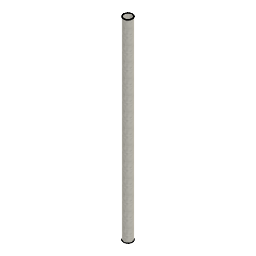
Antenna Assembly (Autodesk Fusion 360 archive; units mm, degrees)
design "GFK Rod"
part number: 2026-07-02-19-40-21-318
Autodesk Fusion 360 part; units mm, degrees
(part 1 of 2)
sketch "Skizze1" plane through (0, 0, 0) normal (0, 0, 1) x (1, 0, 0)
  circle A0 centre (0, 0) radius 14
  circle A1 centre (0, 0) radius 15.5
  dimension "d1" = 28
  dimension "d2" = 31
  constraint coincident A0.centre A1.centre
  measures "d1" diameter of A0
  measures "d2" diameter of A1
extrude "Extrusion1" add sketch "Skizze1" along normal blind 521.6482 and the other way blind 150
equation "d3 = 40 mm + ( 13.25 * 36.2376 ) * 1 mm + 4.5 mm - 3 mm"
named bodies: "GFK Rod"

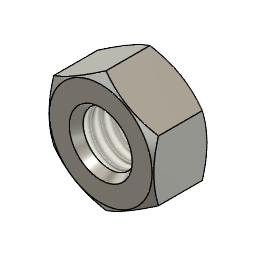
design "Sechskantmutter, normale Form ISO 4032 - M6 Stahl 6 Einfach"
description: Sechskantmutter, normale Form ISO 4032 - M6
part number: ISO 4032 - M6 Stahl 6 Einfach
Autodesk Fusion 360 part; units mm, degrees
sketch "Sketch1" plane through (0, 0, 0) normal (0, 1, 0) x (1, 0, 0)
  line L0 (0, 0) -> (0, -5.2)
  line L1 (-3, 0) -> (-4.9, 0)
  line L2 (-4.9, 0) -> (-5.775, -0.5052)
  line L3 (-5.775, -0.5052) -> (-5.775, -4.6948)
  line L4 (-5.775, -4.6948) -> (-4.9, -5.2)
  line L5 (-4.9, -5.2) -> (-3, -5.2)
  line L6 (-3, -5.2) -> (-3, 0)
  dimension "d121" = 6
  dimension "d122" = 30
  dimension "d123" = 30
  dimension "d128" = 11.55
  dimension "d172" = 9.8
  dimension "d179" = 5.2
  constraint vertical L0
  constraint coincident L0 L0.end
  constraint coincident origin L0
  constraint horizontal L1
  constraint coincident L0.start L1
  constraint coincident L0.start origin
  constraint coincident L0.end L5
  constraint vertical L1.end L4.end
  measures "d122" angle of L1 L2
  measures "d123" angle of L4 L5
  measures "d179" distance of L1 L5
revolve "Revolve1" add sketch "Sketch1" angle 360 about axis through (0, 0, 0) along (0, 0, 1)
sketch "Sketch8" plane through (0, 0, 5.2) normal (0, 0, 1) x (1, 0, 0)
  line L0 (-5, -2.8897) -> (-5, 2.8897)
  circle A0 centre (0, 0) radius 3
  circle A1 centre (0, 0) radius 5.775
  dimension "d114" = 5
  constraint coincident L0.end A1
  constraint coincident L0.start A1
  constraint vertical L0
  measures "d114" distance of A0.centre L0
extrude "Extrude5" cut sketch "Sketch8" against normal blind 5.2 contours L0 A1 picked at (-5.125, -0.7039)
pattern_circular "C-Pattern2" count 6 over 360 about axis through (0, 0, 1.75) along (0, 0, 1) of "Extrude5"
thread "Thread3" "ISO Metric profile 6.0 M6x1 M6x1 6H" major diameter 6.147 minor diameter 5.035 pitch 1 angle 60 resizes the face on face at (-2.9963, 0.1495, 3.4667)
sketch "Sketch12" plane through (0, 0, 0) normal (0, 1, 0) x (1, 0, 0)
  line L0 (-3, 0) -> (0, 0)
  line L1 (-1.4989, -2.6) -> (-3, 0)
  line L2 (-3, -5.2) -> (0, -5.2)
  line L3 (-1.4989, -2.6) -> (-3, -5.2)
  line L4 (0, 0) -> (0, -5.2)
  dimension "d169" = 60
  dimension "d177" = 3
  dimension "d178" = 60
  constraint horizontal L0
  constraint coincident L1.start L3.start
  constraint vertical L0.start L2.start
  constraint coincident L2.end L4.end
  constraint coincident L0.end L4.start
  constraint perpendicular L2 L4
  measures "d169" angle of L2 L3
  measures "d177" distance of L0.start L4
  measures "d178" angle of L0 L1
revolve "Revolve3" cut sketch "Sketch12" angle 360 about axis through (0, 0, 1.75) along (0, 0, 1)
equation "adsk_nheig = 5.20 mm"
equation "adsk_maxdia = 11.55 mm"
equation "adsk_nomdia = 6.00 mm"
equation "d89 = -adsk_nheig"
equation "adsk_waflat = 10.00 mm"
equation "d114 = adsk_waflat / 2"
equation "adsk_chamang1 = 30.00 deg"
equation "adsk_chamang2 = 30.00 deg"
equation "d121 = adsk_nomdia"
equation "d122 = adsk_chamang1"
equation "d123 = adsk_chamang2"
equation "d128 = adsk_maxdia"
equation "d163 = adsk_nheig"
equation "adsk_beardia = 9.80 mm"
equation "d172 = adsk_beardia"
equation "d177 = adsk_nomdia * 0.5"
equation "d179 = adsk_nheig"

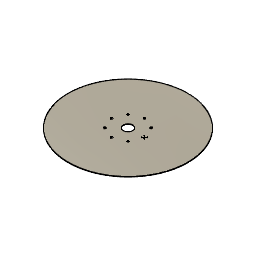
design "Aluminum Reflector"
part number: 2026-07-02-19-35-45-000
Autodesk Fusion 360 part; units mm, degrees
sketch "Skizze1" plane through (0, 0, 0) normal (0, 0, 1) x (1, 0, 0)
  circle A0 centre (0, 0) radius 200
  circle A1 centre (0, 0) radius 15.7
  circle A2 centre (0, 0) radius 54.873
  line L0 (50.553, -4.32) -> (50.553, 4.32)
  circle A3 centre (50.553, -4.32) radius 1.3
  circle A4 centre (59.193, -4.32) radius 1.3
  line L1 (50.553, -4.32) -> (59.193, 4.32) construction
  line L2 (50.553, 4.32) -> (59.193, 4.32)
  line L3 (59.193, -4.32) -> (50.553, 4.32) construction
  line L4 (59.193, 4.32) -> (59.193, -4.32)
  circle A5 centre (50.553, 4.32) radius 1.3
  circle A6 centre (54.873, 0) radius 2.25
  line L5 (59.193, -4.32) -> (50.553, -4.32)
  circle A7 centre (59.193, 4.32) radius 1.3
  circle A8 centre (-54.873, 0) radius 3.1
  circle A9 centre (38.8011, 38.8011) radius 3.1
  circle A10 centre (0, 54.873) radius 3.1
  circle A11 centre (-38.8011, 38.8011) radius 3.1
  circle A12 centre (-38.8011, -38.8011) radius 3.1
  circle A13 centre (0, -54.873) radius 3.1
  circle A14 centre (38.8011, -38.8011) radius 3.1
  point P0 (54.873, 0)
  point P1 (54.873, 0)
  dimension "d1" = 400
  dimension "d2" = 31.4
  dimension "d3" = 109.746
  dimension "d6" = 4.5
  dimension "d7" = 8.64
  dimension "d8" = 8.64
  dimension "d9" = 2.6
  dimension "d10" = 2.6
  dimension "d11" = 2.6
  dimension "d12" = 2.6
  dimension "d13" = 6.2
  dimension "d15" = 270
  constraint coincident A0.centre A1.centre
  constraint concentric A0 A1
  constraint coincident P1 P0
  constraint horizontal L5
  constraint perpendicular L0 L5
  constraint parallel L2 L5
  constraint parallel L0 L4
  constraint coincident P1 L3
  constraint coincident P1 L1
  constraint coincident L1.end L2.end
  constraint coincident A4.centre L3.start
  constraint coincident L0.end L2.start
  constraint coincident L0.start A3.centre
  constraint coincident A2 P1
  constraint horizontal A0.centre P1
  constraint coincident A2 A8.centre
  measures "d1" diameter of A0
  measures "d2" diameter of A1
  measures "d3" diameter of A2
  measures "d6" diameter of A6
  measures "d7" distance of L0.end L1.end
  measures "d8" distance of L0.end L0.start
  measures "d9" diameter of A7
  measures "d10" diameter of A4
  measures "d11" diameter of A5
  measures "d12" diameter of A3
  measures "d13" diameter of A8
extrude "Extrusion1" add sketch "Skizze1" along normal blind 1.5 contours A0 | A2 L0 A3 L2 A5 A6 L5 | A2 A4 L2 L4 A6 L5 A7 | A2 L0 A3 L2 A5 L5 A8 A9 A10 A11 A12 A13 A14
named bodies: "Aluminum Reflector"

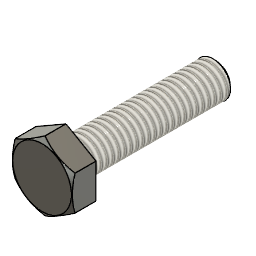
design "Sechskantschraube mit Ganzgewinde DIN EN 24018 - M6 x 25 Stahl 4.6 Einfach"
description: Sechskantschraube mit Ganzgewinde DIN EN 24018 - M6 x 25
part number: DIN EN 24018 - M6 x 25 Stahl 4.6 Einfach
Autodesk Fusion 360 part; units mm, degrees
sketch "Sketch1" plane through (0, 0, 0) normal (0, 1, 0) x (1, 0, 0)
  line L0 (-3, 0) -> (-3, 25)
  line L1 (-3, 25) -> (0, 25)
  line L2 (0, 25) -> (0, -4)
  line L3 (-3, 0) -> (-5.775, 0)
  line L4 (-5.775, 0) -> (-5.775, -3.4948)
  line L5 (-4.9, -4) -> (0, -4)
  line L6 (-5.775, -3.4948) -> (-4.9, -4)
  dimension "d81" = 11.55
  dimension "d135" = 6
  dimension "d137" = 4
  dimension "d138" = 25
  dimension "d153" = 30
  dimension "d154" = 9.8
  constraint perpendicular L0 L1
  constraint perpendicular L0 L3
  constraint coincident origin L3
  constraint vertical L2
  constraint coincident L2 L5.end
  constraint perpendicular L2 L5
  constraint coincident L0.start L3.start
  constraint coincident L0.end L1.start
  constraint coincident origin L2
  constraint vertical L4
  measures "d137" distance of L3 L5
  measures "d138" distance of L1 L3
  measures "d153" angle of L5 L6
revolve "Revolve1" add sketch "Sketch1" angle 360 about axis through (0, 0, -25) along (0, 0, 1)
sketch "Sketch8" plane through (0, 0, 0) normal (0, 0, 1) x (1, 0, 0)
  line L0 (-5, -2.8868) -> (0, -5.7735)
  line L1 (0, -5.7735) -> (5, -2.8868)
  line L2 (5, -2.8868) -> (5, 2.8868)
  line L3 (5, 2.8868) -> (0, 5.7735)
  line L4 (0, 5.7735) -> (-5, 2.8868)
  line L5 (-5, 2.8868) -> (-5, -2.8868)
  circle A0 centre (0, 0) radius 5.8
  dimension "d160" = 10
  dimension "d161" = 11.6
  constraint vertical L5
  constraint coincident A0.centre origin
  measures "d160" distance of L2 L5
  measures "d161" diameter of A0
extrude "Extrude5" cut sketch "Sketch8" along normal through all
thread "Thread3" "ISO Metric profile 6.0 M6x1 M6x1 6g" major diameter 5.884 minor diameter 4.7435 pitch 1 angle 60 resizes the face on face at (-2.9851, 0.2987, -8.3333) from (0, 0, -1) to (0, 0, -25)
sketch "Sketch13" plane through (0, 0, 0) normal (0, 1, 0) x (1, 0, 0)
  line L0 (0, 25) -> (0, -4)
  line L1 (0, 25) -> (-3.06, 25)
  line L2 (-3.06, 25) -> (-3.06, 24.3865)
  line L3 (-3.06, 24.3865) -> (-2.3866, 25)
  dimension "d155" = 0.6135
  dimension "d156" = 2.3866
  dimension "d157" = 3.06
  constraint coincident L0.start L1.start
  constraint perpendicular L0 L1
  constraint perpendicular L1 L2
  constraint coincident L1 L3.end
  measures "d155" distance of L1 L2.end
  measures "d156" distance of L0 L3.end
  measures "d157" distance of L0.start L2
revolve "Revolve4" cut sketch "Sketch13" angle 360 about axis through (0, 0, 1.75) along (0, 0, 1)
equation "adsk_nomlen = 25.00 mm"
equation "adsk_headh = 4.00 mm"
equation "adsk_headdia = 11.55 mm"
equation "adsk_nomdia = 6.00 mm"
equation "d81 = adsk_headdia"
equation "adsk_waflat = 10.00 mm"
equation "adsk_thrlen = 24.00 mm"
equation "adsk_chamang2 = 30.00 deg"
equation "d135 = adsk_nomdia"
equation "d137 = adsk_headh"
equation "d138 = adsk_nomlen"
equation "adsk_endpointdia = 4.7731 mm"
equation "adsk_startlen = 0.61345 mm"
equation "d153 = adsk_chamang2"
equation "d154 = adsk_waflat * 0.98"
equation "d155 = adsk_startlen"
equation "d156 = adsk_endpointdia / 2"
equation "d157 = adsk_nomdia * 0.51"
equation "d159 = min(adsk_thrlen; adsk_nomlen - 0.001 mm)"
equation "d160 = adsk_waflat"
equation "d161 = max(adsk_waflat * 1.16; adsk_headdia)"

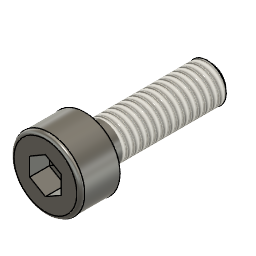
design "Zylinderschraube mit gestanztem Innensechskant ANSI B18.3.1M - M2.5x0.45 x 8 Stahlklasse 2 Einfach"
description: Zylinderschraube mit gestanztem Innensechskant ANSI B18.3.1M - M2.5x0.45 x 8
part number: BSHCS ANSI B18.3.1M - M2.5x0.45 x 8 Stahlklasse 2 Einfach
Autodesk Fusion 360 part; units mm, degrees
sketch "Sketch1" plane through (0, 0, 0) normal (0, 1, 0) x (1, 0, 0)
  line L0 (-1.25, 0) -> (-1.25, 8)
  line L1 (-1.25, 8) -> (0, 8)
  line L2 (0, 8) -> (0, -2.5)
  line L3 (-1.25, 0) -> (-2.25, 0)
  line L4 (-2.25, 0) -> (-2.25, -2.5)
  line L5 (-2.25, -2.5) -> (0, -2.5)
  dimension "d101" = 8
  dimension "d102" = 2.5
  dimension "d109" = 4.5
  dimension "d110" = 2.5
  constraint perpendicular L0 L1
  constraint collinear origin L1.end L2.end
  constraint perpendicular L0 L3
  constraint coincident origin L3
  constraint vertical L2
  constraint coincident L2 L5.end
  constraint perpendicular L2 L5
  measures "d101" distance of origin L1
  measures "d102" distance of L3.end L5
revolve "Revolve1" add sketch "Sketch1" angle 360 about axis through (0, 0, -8) along (0, 0, 1)
ref_plane "WorkPlane1" through (0, 0, 2.5) normal (0, 0, 1) x (1, 0, 0)
sketch "Sketch6" plane through (0, 0, 2.5) normal (0, 0, 1) x (1, 0, 0)
  line L0 (0, -1.1547) -> (1, -0.5774)
  line L1 (1, -0.5774) -> (1, 0.5774)
  line L2 (1, 0.5774) -> (0, 1.1547)
  line L3 (0, 1.1547) -> (-1, 0.5774)
  line L4 (-1, 0.5774) -> (-1, -0.5774)
  line L5 (-1, -0.5774) -> (0, -1.1547)
  dimension "d111" = 2
  constraint vertical L1
  measures "d111" distance of L1 L4
extrude "Extrude1" cut sketch "Sketch6" against normal blind 1.25
extrude "Extrude2" cut 1 faces at (-0.3333, -0.1925, 1.25) along direction (0, 0, -1) blind 1.25 draft -85
thread "Thread3" "ANSI Metric M Profile 2.5 M2.5x0.45 M2.5x0.45 4g6g" major diameter 2.43 minor diameter 1.9295 pitch 0.45 angle 60 resizes the face on face at (-1.2438, 0.1245, -5.3333) from (0, 0, -1.1761) to (0, 0, -8)
fillet "Fillet4" radius 0.25 1 edges at (-2.0977, 0.8136, 2.5)
sketch "Sketch7" plane through (0, 0, 0) normal (0, 1, 0) x (1, 0, 0)
  line L0 (-1.275, 8) -> (-1.275, 7.7239)
  line L1 (-1.275, 7.7239) -> (-0.9739, 8)
  line L2 (0, 8) -> (0, -2.5)
  line L3 (-1.275, 8) -> (0, 8)
  dimension "d104" = 0.9739
  dimension "d105" = 1.275
  dimension "d106" = 0.2761
  constraint coincident L2.start L3.end
  constraint perpendicular L2 L3
  constraint coincident L1.end L3
  constraint perpendicular L0 L3
  measures "d104" distance of L1.end L2
  measures "d105" distance of L0 L2.start
  measures "d106" distance of L0.end L3
revolve "Revolve3" cut sketch "Sketch7" angle 360 about axis through (0, 0, 1.75) along (0, 0, 1)
equation "adsk_nomlen = 8.00 mm"
equation "adsk_headh = 2.50 mm"
equation "adsk_headdia = 4.50 mm"
equation "adsk_nomdia = 2.50 mm"
equation "adsk_philwidth = 2.00 mm"
equation "d31 = -adsk_phildepth"
equation "adsk_phildepth = 1.25 mm"
equation "d71 = adsk_headh"
equation "d76 = -adsk_phildepth"
equation "adsk_thrlen = 6.8239475 mm"
equation "d86 = adsk_nomdia * 0.1"
equation "adsk_startlen = 0.276053 mm"
equation "adsk_endpointdia = 1.947895 mm"
equation "d101 = adsk_nomlen"
equation "d102 = adsk_headh"
equation "d104 = adsk_endpointdia / 2"
equation "d105 = adsk_nomdia * 0.51"
equation "d106 = adsk_startlen"
equation "d108 = min(adsk_thrlen; adsk_nomlen - 0.001 mm)"
equation "d109 = adsk_headdia"
equation "d110 = adsk_nomdia"
equation "d111 = adsk_philwidth"

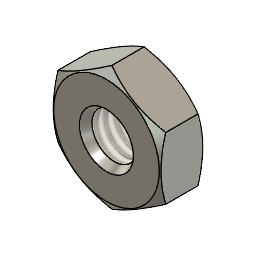
design "Sechskantmutter, normale Form DIN 970 - M2.5 Stahl 6 Einfach"
description: Sechskantmutter, normale Form DIN 970 - M2.5
part number: DIN 970 - M2.5 Stahl 6 Einfach
Autodesk Fusion 360 part; units mm, degrees
sketch "Sketch1" plane through (0, 0, 0) normal (0, 1, 0) x (1, 0, 0)
  line L0 (0, 0) -> (0, -2)
  line L1 (-1.25, 0) -> (-2.45, 0)
  line L2 (-2.45, 0) -> (-2.8875, -0.2526)
  line L3 (-2.8875, -0.2526) -> (-2.8875, -1.7474)
  line L4 (-2.8875, -1.7474) -> (-2.45, -2)
  line L5 (-2.45, -2) -> (-1.25, -2)
  line L6 (-1.25, -2) -> (-1.25, 0)
  dimension "d121" = 2.5
  dimension "d122" = 30
  dimension "d123" = 30
  dimension "d128" = 5.775
  dimension "d172" = 4.9
  dimension "d179" = 2
  constraint vertical L0
  constraint coincident L0 L0.end
  constraint coincident origin L0
  constraint horizontal L1
  constraint coincident L0.start L1
  constraint coincident L0.start origin
  constraint coincident L0.end L5
  constraint vertical L1.end L4.end
  measures "d122" angle of L1 L2
  measures "d123" angle of L4 L5
  measures "d179" distance of L1 L5
revolve "Revolve1" add sketch "Sketch1" angle 360 about axis through (0, 0, 0) along (0, 0, 1)
sketch "Sketch8" plane through (0, 0, 2) normal (0, 0, 1) x (1, 0, 0)
  line L0 (-2.5, -1.4449) -> (-2.5, 1.4449)
  circle A0 centre (0, 0) radius 1.25
  circle A1 centre (0, 0) radius 2.8875
  dimension "d114" = 2.5
  constraint coincident L0.end A1
  constraint coincident L0.start A1
  constraint vertical L0
  measures "d114" distance of A0.centre L0
extrude "Extrude5" cut sketch "Sketch8" against normal blind 2 contours L0 A1 picked at (-2.5625, 0.3519)
pattern_circular "C-Pattern2" count 6 over 360 about axis through (0, 0, 1.75) along (0, 0, 1) of "Extrude5"
thread "Thread3" "ISO Metric profile 2.5 M2.5x0.45 M2.5x0.45 6H" major diameter 2.58 minor diameter 2.0755 pitch 0.45 angle 60 resizes the face on face at (-1.2438, 0.1245, 1.3333)
sketch "Sketch12" plane through (0, 0, 0) normal (0, 1, 0) x (1, 0, 0)
  line L0 (-1.25, 0) -> (0, 0)
  line L1 (-0.6726, -1) -> (-1.25, 0)
  line L2 (-1.25, -2) -> (0, -2)
  line L3 (-0.6726, -1) -> (-1.25, -2)
  line L4 (0, 0) -> (0, -2)
  dimension "d169" = 60
  dimension "d177" = 1.25
  dimension "d178" = 60
  constraint horizontal L0
  constraint coincident L1.start L3.start
  constraint vertical L0.start L2.start
  constraint coincident L2.end L4.end
  constraint coincident L0.end L4.start
  constraint perpendicular L2 L4
  measures "d169" angle of L2 L3
  measures "d177" distance of L0.start L4
  measures "d178" angle of L0 L1
revolve "Revolve3" cut sketch "Sketch12" angle 360 about axis through (0, 0, 1.75) along (0, 0, 1)
equation "adsk_nheig = 2.00 mm"
equation "adsk_maxdia = 5.775 mm"
equation "adsk_nomdia = 2.50 mm"
equation "d89 = -adsk_nheig"
equation "adsk_waflat = 5.00 mm"
equation "d114 = adsk_waflat / 2"
equation "adsk_chamang1 = 30.00 deg"
equation "adsk_chamang2 = 30.00 deg"
equation "d121 = adsk_nomdia"
equation "d122 = adsk_chamang1"
equation "d123 = adsk_chamang2"
equation "d128 = adsk_maxdia"
equation "d163 = adsk_nheig"
equation "adsk_beardia = 4.90 mm"
equation "d172 = adsk_beardia"
equation "d177 = adsk_nomdia * 0.5"
equation "d179 = adsk_nheig"

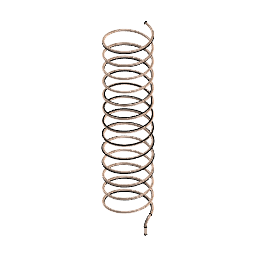
design "Copper Wire"
part number: 2026-07-02-19-25-43-179
Autodesk Fusion 360 part; units mm, degrees
coil "Grundkörper Spirale1" add diameter 109.746 section triangle out size 6 inside turns 13.25 pitch 36.2376 right hand placed x (1, 0, 0) y (0, 1, 0) z (0, 0, 1) at (0, 0, 0) makes body 1
sketch "Skizze2" plane through (0, 0, 0) normal (0, 0, 1) x (1, 0, 0)
  line L0 (54.873, 0, 0) -> (54.873, 0, -20)
  line L1 (54.873, 0, -20) -> (54.873, 0, -40)
  line L2 (54.873, 0, 0) -> (51.2639, 19.5586, 2.1021)
  spline S0 degree 3 poles (51.2639, 19.5586, 2.1021) (50.4481, 21.7028, 2.3432) (49.4982, 23.7958, 2.5844) (48.4186, 25.8203, 2.8255) (44.2021, 33.727, 3.7673) (38.0152, 40.5732, 4.7091) (30.5744, 45.5659, 5.6509) (23.1337, 50.5585, 6.5927) (14.4534, 53.6883, 7.5345) (5.5388, 54.5927, 8.4763) (-3.3756, 55.4972, 9.418) (-12.5073, 54.1747, 10.3598) (-20.7988, 50.7785, 11.3015) (-29.0901, 47.3824, 12.2432) (-36.5255, 41.9191, 13.1849) (-42.2439, 35.0214, 14.1267) (-47.9622, 28.1239, 15.0683) (-51.9527, 19.8051, 16.01) (-53.7534, 11.0283, 16.9517) (-55.554, 2.2518, 17.8934) (-55.1615, -6.966, 18.8351) (-52.6213, -15.5576, 19.7767) (-50.0813, -24.1491, 20.7184) (-45.3985, -32.0981, 21.66) (-39.1152, -38.4844, 22.6016) (-32.8321, -44.8705, 23.5432) (-24.9605, -49.6818, 24.4848) (-16.4118, -52.3612, 25.4264) (-7.8634, -55.0406, 26.368) (1.3459, -55.5832, 27.3096) (10.1498, -53.9261, 28.2512) (18.9535, -52.2691, 29.1927) (27.3351, -48.4158, 30.1343) (34.3244, -42.8122, 31.0758) (41.3134, -37.2088, 32.0173) (46.897, -29.8658, 32.9589) (50.4286, -21.6334, 33.9004) (53.9601, -13.4012, 34.8419) (55.4332, -4.2952, 35.7834) (54.6773, 4.6306, 36.7249) (53.9214, 13.5561, 37.6663) (50.9381, 22.2844, 38.6078) (46.0726, 29.8053, 39.5493) (41.2074, 37.326, 40.4907) (34.4693, 43.625, 41.4322) (26.6384, 47.9734, 42.3736) (18.8077, 52.3215, 43.315) (9.899, 54.7109, 44.2564) (0.9433, 54.8649, 45.1978) (-8.012, 55.0189, 46.1392) (-16.9973, 52.9373, 47.0806) (-24.9727, 48.8611, 48.022) (-32.9479, 44.785, 48.9634) (-39.8981, 38.7222, 49.9047) (-45.019, 31.3741, 50.8461) (-50.1398, 24.0262, 51.7874) (-53.4217, 15.4072, 52.7288) (-54.4849, 6.5143, 53.6701) (-55.5482, -2.3783, 54.6114) (-54.3908, -11.5278, 55.5527) (-51.1469, -19.8756, 56.494) (-47.9031, -28.2232, 57.4353) (-42.5788, -35.7532, 58.3766) (-35.7903, -41.5945, 59.3179) (-29.002, -47.4356, 60.2591) (-20.7622, -51.5769, 61.2004) (-12.0244, -53.5393, 62.1416) (-3.2869, -55.5017, 63.0829) (5.9321, -55.2816, 64.0241) (14.5661, -52.9044, 64.9653) (23.1998, -50.5273, 65.9065) (31.232, -45.9978, 66.8477) (37.7337, -39.8399, 67.7889) (44.2352, -33.6821, 68.7301) (49.1937, -25.9077, 69.6713) (52.0359, -17.416, 70.6125) (54.8779, -8.9245, 71.5536) (55.5982, 0.2682, 72.4948) (54.1134, 9.0988, 73.436) (52.6286, 17.9291, 74.3771) (48.9418, 26.3805, 75.3182) (43.4792, 33.4755, 76.2593) (38.0168, 40.5703, 77.2005) (30.7891, 46.2953, 78.1416) (22.6321, 49.9883, 79.0827) (14.4754, 53.6813, 80.0237) (5.4049, 55.3354, 80.9648) (-3.5303, 54.7593, 81.9059) (-12.4653, 54.1833, 82.847) (-21.2481, 51.3783, 83.788) (-28.863, 46.6688, 84.7291) (-36.4777, 41.9594, 85.6701) (-42.9101, 35.3544, 86.6111) (-47.4163, 27.6178, 87.5522) (-51.9224, 19.8813, 88.4932) (-54.4939, 11.0279, 89.4342) (-54.8335, 2.0812, 90.3752) (-55.1731, -6.8652, 91.3162) (-53.2802, -15.8879, 92.2572) (-49.3736, -23.9435, 93.1982) (-45.4672, -31.9989, 94.1391) (-39.5547, -39.072, 95.0801) (-32.3197, -44.345, 96.021) (-25.0849, -49.6179, 96.962) (-16.5414, -53.0808, 97.9029) (-7.6771, -54.3333, 98.8438) (1.187, -55.5858, 99.7848) (10.3553, -54.6256, 100.7257) (18.7676, -51.5638, 101.6666) (27.5797, -48.3565, 102.6522) (35.542, -42.8457, 103.6378) (41.6478, -35.7282, 104.6235) (47.706, -28.6663, 105.6014) (51.9236, -20.039, 106.5793) (53.7753, -10.9208, 107.5573) (55.6126, -1.8738, 108.5276) (55.1176, 7.6368, 109.4978) (52.3511, 16.4442, 110.4681) (49.6062, 25.1828, 111.4308) (44.6315, 33.211, 112.3935) (38.0283, 39.5588, 113.3563) (31.4766, 45.857, 114.3114) (23.3354, 50.4886, 115.2666) (14.5739, 52.9023, 116.2218) (5.8807, 55.2971, 117.1695) (-3.4059, 55.5045, 118.1173) (-12.1973, 53.5002, 119.065) (-20.9635, 51.5016, 120.01) (-29.2203, 47.3081, 120.955) (-36.0052, 41.4086, 121.9) (-42.7894, 35.5096, 122.8449) (-48.089, 27.9163, 123.7898) (-51.286, 19.5138, 124.7347) (-54.4828, 11.112, 125.6795) (-55.5714, 1.9174, 126.6244) (-54.4249, -6.9986, 127.5692) (-53.2785, -15.9137, 128.5139) (-49.8996, -24.533, 129.4587) (-44.682, -31.8522, 130.4034) (-39.4649, -39.1707, 131.348) (-32.4194, -45.1753, 132.2927) (-24.3664, -49.1663, 133.2373) (-16.3142, -53.1569, 134.1819) (-7.27, -55.1267, 135.1265) (1.7125, -54.8463, 136.071) (10.6942, -54.5658, 137.0155) (19.597, -52.0361, 137.96) (27.3842, -47.5516, 138.9044) (35.1706, -43.0675, 139.8488) (41.8265, -36.6377, 140.7932) (46.577, -29.0109, 141.7376) (51.327, -21.3848, 142.6819) (54.1627, -12.5764, 143.6262) (54.754, -3.6114, 144.5705) (55.3453, 5.3528, 145.5148) (53.6914, 14.4564, 146.459) (49.9848, 22.6398, 147.4032) (46.2786, 30.8225, 148.3474) (40.5272, 38.0694, 149.2915) (33.4001, 43.5371, 150.2356) (26.2735, 49.0044, 151.1797) (17.7851, 52.6822, 152.1238) (8.9225, 54.1427, 153.0678) (0.0607, 55.6031, 154.0118) (-9.1583, 54.8438, 154.9558) (-17.6617, 51.953, 155.8998) (-26.1644, 49.0624, 156.8437) (-33.9354, 44.0464, 157.7876) (-40.0708, 37.4884, 158.7315) (-46.2057, 30.9309, 159.6753) (-50.6934, 22.8442, 160.6191) (-53.0121, 14.1689, 161.5629) (-55.3307, 5.4944, 162.5067) (-55.476, -3.7522, 163.4504) (-53.4314, -12.4953, 164.3941) (-51.3869, -21.2378, 165.3378) (-47.1566, -29.4603, 166.2815) (-41.2325, -36.2067, 167.2251) (-35.3088, -42.9527, 168.1687) (-27.7029, -48.2099, 169.1123) (-19.2988, -51.3673, 170.0559) (-10.8954, -54.5245, 170.9994) (-1.7102, -55.5761, 171.9429) (7.1893, -54.4, 172.8864) (16.088, -53.224, 173.8298) (24.6841, -49.8228, 174.7733) (31.9784, -44.5918, 175.7167) (39.2722, -39.3611, 176.6601) (45.2505, -32.3109, 177.6034) (49.2187, -24.2604, 178.5468) (53.1866, -16.2104, 179.4901) (55.1371, -7.1757, 180.4333) (54.8437, 1.7942, 181.3766) (54.5502, 10.7635, 182.3198) (52.0137, 19.6507, 183.263) (47.5288, 27.4237, 184.2062) (43.0443, 35.196, 185.1494) (36.6202, 41.8393, 186.0925) (29.0026, 46.5821, 187.0356) (21.3857, 51.3245, 187.9787) (12.5901, 54.1576, 188.9218) (3.6372, 54.7523, 189.8648) (-5.315, 55.347, 190.8078) (-14.4074, 53.7026, 191.7508) (-22.5842, 50.01, 192.6938) (-30.7604, 46.3177, 193.6367) (-38.0056, 40.5845, 194.5796) (-43.4787, 33.4761, 195.5226) (-48.9513, 26.3682, 196.4654) (-52.6417, 17.8989, 197.4083) (-54.1214, 9.0512, 198.3511) (-55.6009, 0.2041, 199.2939) (-54.8673, -9.0044, 200.2367) (-52.0057, -17.5057, 201.1795) (-49.1443, -26.0063, 202.1222) (-44.1607, -33.7835, 203.0649) (-37.6331, -39.9349, 204.0076) (-31.106, -46.0858, 204.9502) (-23.0477, -50.5993, 205.8929) (-14.3931, -52.9517, 206.8355) (-5.7391, -55.304, 207.7781) (3.4946, -55.4911, 208.7207) (12.2368, -53.4912, 209.6632) (20.9783, -51.4915, 210.6058) (29.2118, -47.3089, 211.5483) (35.9821, -41.4287, 212.4908) (42.7519, -35.5489, 213.4332) (48.0459, -27.9829, 214.3757) (51.25, -19.6082, 215.3181) (54.4539, -11.2341, 216.2605) (55.5622, -2.0673, 217.2029) (54.4464, 6.8291, 218.1452) (53.3306, 15.7249, 219.0875) (49.9931, 24.3334, 220.0299) (44.8209, 31.6565, 220.9722) (39.649, 38.9791, 221.9144) (32.6524, 45.0026, 222.8567) (24.6424, 49.0285, 223.7989) (16.6329, 53.0542, 224.7411) (7.6252, 55.075, 225.6833) (-1.3364, 54.8567, 226.6255) (-10.2974, 54.6384, 227.5676) (-19.1954, 52.1817, 228.5097) (-26.999, 47.7713, 229.4518) (-34.8021, 43.3612, 230.3939) (-41.4962, 37.0061, 231.336) (-46.3054, 29.4425, 232.278) (-51.1143, 21.8793, 233.22) (-54.0294, 13.1222, 234.162) (-54.7131, 4.1858, 235.104) (-55.3967, -4.7501, 236.046) (-53.8479, -13.8482, 236.9879) (-50.2459, -22.0544, 237.9298) (-46.6442, -30.2601, 238.8717) (-40.9965, -37.5585, 239.8136) (-33.9571, -43.1041, 240.7555) (-26.9181, -48.6493, 241.6973) (-18.501, -52.4314, 242.6391) (-9.6808, -54.0123, 243.581) (-0.8611, -55.5931, 244.5227) (8.345, -54.9699, 245.4645) (16.8713, -52.215, 246.4062) (25.397, -49.4602, 247.3479) (33.2267, -44.5792, 248.2897) (39.4538, -38.1372, 249.2314) (45.6805, -31.6955, 250.173) (50.2929, -23.7052, 251.1147) (52.7569, -15.0915, 252.0563) (55.2208, -6.4784, 252.9979) (55.5318, 2.7418, 253.9395) (53.6541, 11.5014, 254.8811) (51.7765, 20.2606, 255.8226) (47.7139, 28.5426, 256.7642) (41.9366, 35.3888, 257.7057) (36.1596, 42.2347, 258.6472) (28.6791, 47.6318, 259.5887) (20.361, 50.9556, 260.5301) (12.0434, 54.2792, 261.4716) (2.904, 55.5233, 262.413) (-5.9994, 54.5441, 263.3544) (-14.9023, 53.5648, 264.2958) (-23.5523, 50.3642, 265.2372) (-30.9484, 45.3127, 266.1785) (-38.3441, 40.2615, 267.1199) (-44.472, 33.3691, 268.0612) (-48.6231, 25.4331, 269.0025) (-52.7739, 17.4976, 269.9438) (-54.9402, 8.5336, 270.8851) (-54.8714, -0.4217, 271.8263) (-54.8026, -9.3765, 272.7675) (-52.499, -18.3057, 273.7088) (-48.2271, -26.1762, 274.65) (-43.9555, -34.0463, 275.5911) (-37.7238, -40.8429, 276.5323) (-30.2531, -45.7798, 277.4735) (-22.7828, -50.7165, 278.4146) (-14.0877, -53.7844, 279.3557) (-5.1734, -54.6286, 280.2968) (3.7404, -55.4727, 281.2379) (12.8563, -54.0919, 282.179) (21.1202, -50.6457, 283.12) (29.3837, -47.1996, 284.0611) (36.7795, -41.695, 285.0021) (42.4524, -34.7684, 285.9431) (48.125, -27.8421, 286.8841) (52.0641, -19.5071, 287.8251) (53.8143, -10.7271, 288.766) (55.5644, -1.9475, 289.707) (55.1224, 7.2604, 290.6479) (52.5395, 15.832, 291.5888) (49.8436, 24.7785, 292.5709) (44.8171, 33.0118, 293.553) (38.0914, 39.498, 294.535) (31.4707, 45.8829, 295.5018) (23.2186, 50.5623, 296.4685) (14.3404, 52.966, 297.4353) (5.6009, 55.3322, 298.3869) (-3.7272, 55.4899, 299.3385) (-12.5417, 53.4205, 300.2901) (-21.2944, 51.3656, 301.2351) (-29.5237, 47.1193, 302.1801) (-36.2702, 41.1766, 303.125) (-43.0156, 35.2351, 304.0698) (-48.2657, 27.6092, 305.0146) (-51.4089, 19.1877, 305.9594) (-54.5516, 10.7677, 306.904) (-55.582, 1.5686, 307.8486) (-54.3801, -7.338, 308.7932) (-53.1785, -16.243, 309.7376) (-49.7478, -24.8384, 310.682) (-44.4874, -32.1234, 311.6265) (-39.228, -39.4072, 312.5707) (-32.1497, -45.3669, 313.515) (-24.0766, -49.3088, 314.4593) (-16.005, -53.2501, 315.4034) (-6.9543, -55.1667, 316.3475) (2.0222, -54.8357, 317.2916) (10.997, -54.5048, 318.2355) (19.8805, -51.9276, 319.1795) (27.639, -47.4039, 320.1234) (35.3962, -42.8811, 321.0672) (42.0141, -36.4211, 322.011) (46.7229, -28.7753, 322.9548) (51.4309, -21.1308, 323.8984) (54.2216, -12.3155, 324.842) (54.7704, -3.3543, 325.7856) (55.3191, 5.6054, 326.7291) (53.6257, 14.6938, 327.6726) (49.887, 22.8547, 328.616) (46.1488, 31.0143, 329.5594) (40.3732, 38.2309, 330.5027) (33.2311, 43.6663, 331.446) (26.0901, 49.1007, 332.3892) (17.5967, 52.744, 333.3323) (8.7376, 54.1729, 334.2755) (-0.1203, 55.6016, 335.2185) (-9.3269, 54.8138, 336.1616) (-17.8133, 51.9012, 337.1046) (-26.2984, 48.989, 338.0475) (-34.0472, 43.958, 338.9904) (-40.1604, 37.3924, 339.9333) (-46.2726, 30.8277, 340.876) (-50.7379, 22.7413, 341.8188) (-53.0381, 14.0716, 342.7615) (-55.3379, 5.4032, 343.7041) (-55.4689, -3.8318, 344.6467) (-53.4158, -12.562, 345.5893) (-51.3629, -21.2909, 346.5318) (-47.1306, -29.4985, 347.4743) (-41.2097, -36.2327, 348.4168) (-35.2895, -42.9661, 349.3591) (-27.6925, -48.2137, 350.3015) (-19.2995, -51.3671, 351.2438) (-10.9077, -54.52, 352.186) (-1.7361, -55.5733, 353.1282) (7.152, -54.4049, 354.0705) (16.039, -53.2366, 355.0125) (24.6256, -49.8494, 355.9546) (31.9168, -44.6359, 356.8967) (39.2071, -39.423, 357.8387) (45.1883, -32.3942, 358.7807) (49.1676, -24.3638, 359.7226) (53.1464, -16.3344, 360.6645) (55.1161, -7.319, 361.6064) (54.8485, 1.6381, 362.5482) (54.5811, 10.5941, 363.4899) (52.0774, 19.4749, 364.4317) (47.6276, 27.2518, 365.3734) (43.1783, 35.0278, 366.315) (36.7917, 41.6855, 367.2566) (29.2073, 46.454, 368.1983) (21.6238, 51.2221, 369.1398) (12.8572, 54.0923, 370.0813) (3.9223, 54.7326, 371.0228) (-5.0117, 55.3729, 371.9642) (-14.0969, 53.7824, 372.9056) (-22.2821, 50.1453, 373.847) (-30.4663, 46.5087, 374.7883) (-37.7351, 40.8328, 375.7296) (-43.2474, 33.7744, 376.6709) (-48.7591, 26.7167, 377.6121) (-52.5043, 18.2902, 378.5533) (-54.0497, 9.4697, 379.4945) (-55.5949, 0.6502, 380.4356) (-54.9379, -8.5466, 381.3767) (-52.1546, -17.057, 382.3178) (-49.3717, -25.5664, 383.2588) (-44.4681, -33.3735, 384.1998) (-38.0111, -39.5753, 385.1408) (-31.2201, -46.0978, 386.1304) (-22.7221, -50.8273, 387.1201) (-13.5999, -53.161, 388.1097) (-4.7627, -55.4217, 389.0685) (4.6405, -55.4321, 390.0272) (13.4826, -53.1908, 390.9859) (22.1968, -50.982, 391.9308) (30.3491, -46.5918, 392.8757) (36.9893, -40.5319, 393.8205) (43.6272, -34.4742, 394.765) (48.7413, -26.7598, 395.7096) (51.7361, -18.2871, 396.6541) (54.7299, -9.8174, 397.5982) (55.6002, -0.6062, 398.5424) (54.2456, 8.2743, 399.4866) (52.8914, 17.1518, 400.4305) (49.3167, 25.6818, 401.3743) (43.937, 32.8723, 402.3182) (38.5591, 40.0603, 403.2617) (31.3879, 45.8959, 404.2052) (23.2569, 49.7007, 405.1488) (15.1285, 53.5043, 406.092) (6.0564, 55.2712, 407.0353) (-2.9053, 54.796, 407.9785) (-11.8643, 54.321, 408.9215) (-20.6959, 51.6063, 409.8644) (-28.3749, 46.9671, 410.8074) (-36.0516, 42.3293, 411.75) (-42.5617, 35.7769, 412.6927) (-47.1498, 28.0704, 413.6354) (-51.7365, 20.366, 414.5778) (-54.3936, 11.5227, 415.5202) (-54.813, 2.5661, 416.4626) (-55.2322, -6.388, 417.4047) (-53.414, -15.4383, 418.3469) (-49.5692, -23.5359, 419.289) (-45.7255, -31.6313, 420.2309) (-39.8634, -38.759, 421.1729) (-32.6623, -44.0933, 422.1148) (-25.4629, -49.4263, 423.0564) (-16.9388, -52.9565, 423.9981) (-8.077, -54.2753, 424.9398) (0.7827, -55.5938, 425.8812) (9.9632, -54.6993, 426.8227) (18.4018, -51.6955, 427.7641) (26.8385, -48.6923, 428.7054) (34.5177, -43.5864, 429.6466) (40.551, -36.9684, 430.5879) (46.583, -30.3519, 431.5289) (50.9583, -22.2365, 432.4699) (53.171, -13.5608, 433.411) (55.4604, -4.5841, 434.3847) (55.4267, 4.9747, 435.3584) (53.0741, 13.935, 436.3321) (50.7916, 22.6283, 437.2767) (46.3335, 30.7415, 438.2214) (40.2191, 37.3292, 439.1661) (34.1091, 43.9122, 440.1101) (26.357, 48.9594, 441.0541) (17.8648, 51.8835, 441.9981) (9.3782, 54.8056, 442.9414) (0.1687, 55.602, 443.8848) (-8.6936, 54.18, 444.8282) (-17.5504, 52.7588, 445.771) (-26.0435, 49.1248, 446.7138) (-33.1871, 43.6997, 447.6566) (-40.3267, 38.2776, 448.5989) (-46.1047, 31.0768, 449.5411) (-49.8514, 22.9322, 450.4834) (-53.5961, 14.7918, 451.4252) (-55.3043, 5.724, 452.367) (-54.7784, -3.221, 453.3087) (-54.2527, -12.1617, 454.2501) (-51.4958, -20.9628, 455.1914) (-46.8269, -28.6057, 456.1327) (-42.1599, -36.2454, 457.0737) (-35.5913, -42.7136, 458.0146) (-27.8806, -47.2622, 458.9556) (-20.1421, -51.8273, 459.8999) (-11.2678, -54.45, 460.8442) (-2.291, -54.8252, 461.7885) (6.674, -55.1998, 462.7316) (15.7241, -53.3321, 463.6747) (23.8083, -49.439, 464.6178) (31.8834, -45.5503, 465.5598) (38.9794, -39.6482, 466.5018) (44.2742, -32.4167, 467.4438) (49.564, -25.192, 468.3849) (53.0459, -16.6541, 469.3261) (54.3172, -7.7906, 470.2672) (55.5919, 1.0969, 471.2109) (54.6413, 10.2949, 472.1546) (51.576, 18.7339, 473.0982) (48.5177, 27.1538, 474.0398) (43.3601, 34.8023, 474.9813) (36.7004, 40.7937, 475.9229) (30.0339, 46.7913, 476.8654) (21.8748, 51.117, 477.8079) (13.1696, 53.2692, 478.7504) (8.866, 54.3332, 479.2163) (4.4331, 54.873, 479.6823) (0, 54.873, 480.1482) knots 0.36447305 0.36447305 0.36447305 0.36447305 0.48991047 0.48991047 0.48991047 0.9798057 0.9798057 0.9798057 1.46968578 1.46968578 1.46968578 1.95955079 1.95955079 1.95955079 2.44940083 2.44940083 2.44940083 2.93923599 2.93923599 2.93923599 3.42905636 3.42905636 3.42905636 3.91886203 3.91886203 3.91886203 4.4086531 4.4086531 4.4086531 4.89842966 4.89842966 4.89842966 5.38819179 5.38819179 5.38819179 5.87793959 5.87793959 5.87793959 6.36767314 6.36767314 6.36767314 6.85739255 6.85739255 6.85739255 7.3470979 7.3470979 7.3470979 7.83678928 7.83678928 7.83678928 8.32646678 8.32646678 8.32646678 8.8161305 8.8161305 8.8161305 9.30578053 9.30578053 9.30578053 9.79541695 9.79541695 9.79541695 10.28503986 10.28503986 10.28503986 10.77464934 10.77464934 10.77464934 11.2642455 11.2642455 11.2642455 11.75382841 11.75382841 11.75382841 12.24339818 12.24339818 12.24339818 12.73295489 12.73295489 12.73295489 13.22249863 13.22249863 13.22249863 13.7120295 13.7120295 13.7120295 14.20154757 14.20154757 14.20154757 14.69105296 14.69105296 14.69105296 15.18054574 15.18054574 15.18054574 15.670026 15.670026 15.670026 16.15949384 16.15949384 16.15949384 16.64894935 16.64894935 16.64894935 17.13839262 17.13839262 17.13839262 17.62782374 17.62782374 17.62782374 18.14051422 18.14051422 18.14051422 18.64919931 18.64919931 18.64919931 19.15391029 19.15391029 19.15391029 19.65467822 19.65467822 19.65467822 20.1515339 20.1515339 20.1515339 20.6445079 20.6445079 20.6445079 21.13606412 21.13606412 21.13606412 21.62757405 21.62757405 21.62757405 22.11903806 22.11903806 22.11903806 22.61045653 22.61045653 22.61045653 23.10182983 23.10182983 23.10182983 23.59315835 23.59315835 23.59315835 24.08444246 24.08444246 24.08444246 24.57568254 24.57568254 24.57568254 25.06687896 25.06687896 25.06687896 25.5580321 25.5580321 25.5580321 26.04914234 26.04914234 26.04914234 26.54021005 26.54021005 26.54021005 27.0312356 27.0312356 27.0312356 27.52221938 27.52221938 27.52221938 28.01316175 28.01316175 28.01316175 28.50406309 28.50406309 28.50406309 28.99492377 28.99492377 28.99492377 29.48574417 29.48574417 29.48574417 29.97652466 29.97652466 29.97652466 30.46726561 30.46726561 30.46726561 30.95796739 30.95796739 30.95796739 31.44863038 31.44863038 31.44863038 31.93925495 31.93925495 31.93925495 32.42984148 32.42984148 32.42984148 32.92039032 32.92039032 32.92039032 33.41090185 33.41090185 33.41090185 33.90137645 33.90137645 33.90137645 34.39181448 34.39181448 34.39181448 34.88221631 34.88221631 34.88221631 35.37258232 35.37258232 35.37258232 35.86291287 35.86291287 35.86291287 36.35320833 36.35320833 36.35320833 36.84346907 36.84346907 36.84346907 37.33369547 37.33369547 37.33369547 37.82388788 37.82388788 37.82388788 38.31404667 38.31404667 38.31404667 38.80417222 38.80417222 38.80417222 39.2942649 39.2942649 39.2942649 39.78432506 39.78432506 39.78432506 40.27435308 40.27435308 40.27435308 40.76434932 40.76434932 40.76434932 41.25431415 41.25431415 41.25431415 41.74424793 41.74424793 41.74424793 42.23415104 42.23415104 42.23415104 42.72402384 42.72402384 42.72402384 43.21386669 43.21386669 43.21386669 43.70367996 43.70367996 43.70367996 44.19346402 44.19346402 44.19346402 44.68321922 44.68321922 44.68321922 45.17294594 45.17294594 45.17294594 45.66264454 45.66264454 45.66264454 46.15231538 46.15231538 46.15231538 46.64195883 46.64195883 46.64195883 47.13157525 47.13157525 47.13157525 47.621165 47.621165 47.621165 48.11072845 48.11072845 48.11072845 48.60026597 48.60026597 48.60026597 49.08977791 49.08977791 49.08977791 49.57926463 49.57926463 49.57926463 50.06872651 50.06872651 50.06872651 50.5581639 50.5581639 50.5581639 51.0690083 51.0690083 51.0690083 51.57187075 51.57187075 51.57187075 52.06687598 52.06687598 52.06687598 52.55840983 52.55840983 52.55840983 53.04985183 53.04985183 53.04985183 53.54120348 53.54120348 53.54120348 54.0324663 54.0324663 54.0324663 54.52364179 54.52364179 54.52364179 55.01473145 55.01473145 55.01473145 55.50573679 55.50573679 55.50573679 55.9966593 55.9966593 55.9966593 56.48750049 56.48750049 56.48750049 56.97826183 56.97826183 56.97826183 57.46894483 57.46894483 57.46894483 57.95955097 57.95955097 57.95955097 58.45008174 58.45008174 58.45008174 58.94053862 58.94053862 58.94053862 59.43092308 59.43092308 59.43092308 59.92123662 59.92123662 59.92123662 60.41148071 60.41148071 60.41148071 60.90165682 60.90165682 60.90165682 61.39176642 61.39176642 61.39176642 61.88181099 61.88181099 61.88181099 62.37179199 62.37179199 62.37179199 62.86171089 62.86171089 62.86171089 63.35156915 63.35156915 63.35156915 63.84136823 63.84136823 63.84136823 64.3311096 64.3311096 64.3311096 64.82079472 64.82079472 64.82079472 65.31042503 65.31042503 65.31042503 65.80000201 65.80000201 65.80000201 66.28952709 66.28952709 66.28952709 66.77900174 66.77900174 66.77900174 67.29378935 67.29378935 67.29378935 67.79248985 67.79248985 67.79248985 68.28397383 68.28397383 68.28397383 68.77527722 68.77527722 68.77527722 69.26640607 69.26640607 69.26640607 69.75736637 69.75736637 69.75736637 70.24816413 70.24816413 70.24816413 70.7388053 70.7388053 70.7388053 71.22929584 71.22929584 71.22929584 71.71964167 71.71964167 71.71964167 72.20984871 72.20984871 72.20984871 72.69992286 72.69992286 72.69992286 73.18986999 73.18986999 73.18986999 73.67969595 73.67969595 73.67969595 74.16940661 74.16940661 74.16940661 74.65900779 74.65900779 74.65900779 75.14850531 75.14850531 75.14850531 75.65498656 75.65498656 75.65498656 76.14637232 76.14637232 76.14637232 76.6374094 76.6374094 76.6374094 77.1281218 77.1281218 77.1281218 77.61853336 77.61853336 77.61853336 78.10866777 78.10866777 78.10866777 78.59854859 78.59854859 78.59854859 79.08819924 79.08819924 79.08819924 79.57764303 79.57764303 79.57764303 80.06884977 80.06884977 80.06884977 80.55940713 80.55940713 80.55940713 81.04941027 81.04941027 81.04941027 81.53895323 81.53895323 81.53895323 82.02982017 82.02982017 82.02982017 82.51957875 82.51957875 82.51957875 83.00983873 83.00983873 83.00983873 83.25220532 83.25220532 83.25220532 83.25220532
  line L3 (51.2639, 19.5586, 2.1021) -> (50.4481, 21.7028, 2.3432) construction
  line L4 (50.4481, 21.7028, 2.3432) -> (49.4982, 23.7958, 2.5844) construction
  line L5 (49.4982, 23.7958, 2.5844) -> (48.4186, 25.8203, 2.8255) construction
  line L6 (48.4186, 25.8203, 2.8255) -> (44.2021, 33.727, 3.7673) construction
  line L7 (44.2021, 33.727, 3.7673) -> (38.0152, 40.5732, 4.7091) construction
  line L8 (38.0152, 40.5732, 4.7091) -> (30.5744, 45.5659, 5.6509) construction
  line L9 (30.5744, 45.5659, 5.6509) -> (23.1337, 50.5585, 6.5927) construction
  line L10 (23.1337, 50.5585, 6.5927) -> (14.4534, 53.6883, 7.5345) construction
  line L11 (14.4534, 53.6883, 7.5345) -> (5.5388, 54.5927, 8.4763) construction
  line L12 (5.5388, 54.5927, 8.4763) -> (-3.3756, 55.4972, 9.418) construction
  line L13 (-3.3756, 55.4972, 9.418) -> (-12.5073, 54.1747, 10.3598) construction
  line L14 (-12.5073, 54.1747, 10.3598) -> (-20.7988, 50.7785, 11.3015) construction
  line L15 (-20.7988, 50.7785, 11.3015) -> (-29.0901, 47.3824, 12.2432) construction
  line L16 (-29.0901, 47.3824, 12.2432) -> (-36.5255, 41.9191, 13.1849) construction
  line L17 (-36.5255, 41.9191, 13.1849) -> (-42.2439, 35.0214, 14.1267) construction
  line L18 (-42.2439, 35.0214, 14.1267) -> (-47.9622, 28.1239, 15.0683) construction
  line L19 (-47.9622, 28.1239, 15.0683) -> (-51.9527, 19.8051, 16.01) construction
  line L20 (-51.9527, 19.8051, 16.01) -> (-53.7534, 11.0283, 16.9517) construction
  line L21 (-53.7534, 11.0283, 16.9517) -> (-55.554, 2.2518, 17.8934) construction
  line L22 (-55.554, 2.2518, 17.8934) -> (-55.1615, -6.966, 18.8351) construction
  line L23 (-55.1615, -6.966, 18.8351) -> (-52.6213, -15.5576, 19.7767) construction
  line L24 (-52.6213, -15.5576, 19.7767) -> (-50.0813, -24.1491, 20.7184) construction
  line L25 (-50.0813, -24.1491, 20.7184) -> (-45.3985, -32.0981, 21.66) construction
  line L26 (-45.3985, -32.0981, 21.66) -> (-39.1152, -38.4844, 22.6016) construction
  line L27 (-39.1152, -38.4844, 22.6016) -> (-32.8321, -44.8705, 23.5432) construction
  line L28 (-32.8321, -44.8705, 23.5432) -> (-24.9605, -49.6818, 24.4848) construction
  line L29 (-24.9605, -49.6818, 24.4848) -> (-16.4118, -52.3612, 25.4264) construction
  line L30 (-16.4118, -52.3612, 25.4264) -> (-7.8634, -55.0406, 26.368) construction
  line L31 (-7.8634, -55.0406, 26.368) -> (1.3459, -55.5832, 27.3096) construction
  line L32 (1.3459, -55.5832, 27.3096) -> (10.1498, -53.9261, 28.2512) construction
  line L33 (10.1498, -53.9261, 28.2512) -> (18.9535, -52.2691, 29.1927) construction
  line L34 (18.9535, -52.2691, 29.1927) -> (27.3351, -48.4158, 30.1343) construction
  line L35 (27.3351, -48.4158, 30.1343) -> (34.3244, -42.8122, 31.0758) construction
  line L36 (34.3244, -42.8122, 31.0758) -> (41.3134, -37.2088, 32.0173) construction
  line L37 (41.3134, -37.2088, 32.0173) -> (46.897, -29.8658, 32.9589) construction
  line L38 (46.897, -29.8658, 32.9589) -> (50.4286, -21.6334, 33.9004) construction
  line L39 (50.4286, -21.6334, 33.9004) -> (53.9601, -13.4012, 34.8419) construction
  line L40 (53.9601, -13.4012, 34.8419) -> (55.4332, -4.2952, 35.7834) construction
  line L41 (55.4332, -4.2952, 35.7834) -> (54.6773, 4.6306, 36.7249) construction
  line L42 (54.6773, 4.6306, 36.7249) -> (53.9214, 13.5561, 37.6663) construction
  line L43 (53.9214, 13.5561, 37.6663) -> (50.9381, 22.2844, 38.6078) construction
  line L44 (50.9381, 22.2844, 38.6078) -> (46.0726, 29.8053, 39.5493) construction
  line L45 (46.0726, 29.8053, 39.5493) -> (41.2074, 37.326, 40.4907) construction
  line L46 (41.2074, 37.326, 40.4907) -> (34.4693, 43.625, 41.4322) construction
  line L47 (34.4693, 43.625, 41.4322) -> (26.6384, 47.9734, 42.3736) construction
  line L48 (26.6384, 47.9734, 42.3736) -> (18.8077, 52.3215, 43.315) construction
  line L49 (18.8077, 52.3215, 43.315) -> (9.899, 54.7109, 44.2564) construction
  line L50 (9.899, 54.7109, 44.2564) -> (0.9433, 54.8649, 45.1978) construction
  line L51 (0.9433, 54.8649, 45.1978) -> (-8.012, 55.0189, 46.1392) construction
  line L52 (-8.012, 55.0189, 46.1392) -> (-16.9973, 52.9373, 47.0806) construction
  line L53 (-16.9973, 52.9373, 47.0806) -> (-24.9727, 48.8611, 48.022) construction
  line L54 (-24.9727, 48.8611, 48.022) -> (-32.9479, 44.785, 48.9634) construction
  line L55 (-32.9479, 44.785, 48.9634) -> (-39.8981, 38.7222, 49.9047) construction
  line L56 (-39.8981, 38.7222, 49.9047) -> (-45.019, 31.3741, 50.8461) construction
  line L57 (-45.019, 31.3741, 50.8461) -> (-50.1398, 24.0262, 51.7874) construction
  line L58 (-50.1398, 24.0262, 51.7874) -> (-53.4217, 15.4072, 52.7288) construction
  line L59 (-53.4217, 15.4072, 52.7288) -> (-54.4849, 6.5143, 53.6701) construction
  line L60 (-54.4849, 6.5143, 53.6701) -> (-55.5482, -2.3783, 54.6114) construction
  line L61 (-55.5482, -2.3783, 54.6114) -> (-54.3908, -11.5278, 55.5527) construction
  line L62 (-54.3908, -11.5278, 55.5527) -> (-51.1469, -19.8756, 56.494) construction
  line L63 (-51.1469, -19.8756, 56.494) -> (-47.9031, -28.2232, 57.4353) construction
  line L64 (-47.9031, -28.2232, 57.4353) -> (-42.5788, -35.7532, 58.3766) construction
  line L65 (-42.5788, -35.7532, 58.3766) -> (-35.7903, -41.5945, 59.3179) construction
  line L66 (-35.7903, -41.5945, 59.3179) -> (-29.002, -47.4356, 60.2591) construction
  line L67 (-29.002, -47.4356, 60.2591) -> (-20.7622, -51.5769, 61.2004) construction
  line L68 (-20.7622, -51.5769, 61.2004) -> (-12.0244, -53.5393, 62.1416) construction
  line L69 (-12.0244, -53.5393, 62.1416) -> (-3.2869, -55.5017, 63.0829) construction
  line L70 (-3.2869, -55.5017, 63.0829) -> (5.9321, -55.2816, 64.0241) construction
  line L71 (5.9321, -55.2816, 64.0241) -> (14.5661, -52.9044, 64.9653) construction
  line L72 (14.5661, -52.9044, 64.9653) -> (23.1998, -50.5273, 65.9065) construction
  line L73 (23.1998, -50.5273, 65.9065) -> (31.232, -45.9978, 66.8477) construction
  line L74 (31.232, -45.9978, 66.8477) -> (37.7337, -39.8399, 67.7889) construction
  line L75 (37.7337, -39.8399, 67.7889) -> (44.2352, -33.6821, 68.7301) construction
  line L76 (44.2352, -33.6821, 68.7301) -> (49.1937, -25.9077, 69.6713) construction
  line L77 (49.1937, -25.9077, 69.6713) -> (52.0359, -17.416, 70.6125) construction
  line L78 (52.0359, -17.416, 70.6125) -> (54.8779, -8.9245, 71.5536) construction
  line L79 (54.8779, -8.9245, 71.5536) -> (55.5982, 0.2682, 72.4948) construction
  line L80 (55.5982, 0.2682, 72.4948) -> (54.1134, 9.0988, 73.436) construction
  line L81 (54.1134, 9.0988, 73.436) -> (52.6286, 17.9291, 74.3771) construction
  line L82 (52.6286, 17.9291, 74.3771) -> (48.9418, 26.3805, 75.3182) construction
  line L83 (48.9418, 26.3805, 75.3182) -> (43.4792, 33.4755, 76.2593) construction
  line L84 (43.4792, 33.4755, 76.2593) -> (38.0168, 40.5703, 77.2005) construction
  line L85 (38.0168, 40.5703, 77.2005) -> (30.7891, 46.2953, 78.1416) construction
  line L86 (30.7891, 46.2953, 78.1416) -> (22.6321, 49.9883, 79.0827) construction
  line L87 (22.6321, 49.9883, 79.0827) -> (14.4754, 53.6813, 80.0237) construction
  line L88 (14.4754, 53.6813, 80.0237) -> (5.4049, 55.3354, 80.9648) construction
  line L89 (5.4049, 55.3354, 80.9648) -> (-3.5303, 54.7593, 81.9059) construction
  line L90 (-3.5303, 54.7593, 81.9059) -> (-12.4653, 54.1833, 82.847) construction
  line L91 (-12.4653, 54.1833, 82.847) -> (-21.2481, 51.3783, 83.788) construction
  line L92 (-21.2481, 51.3783, 83.788) -> (-28.863, 46.6688, 84.7291) construction
  line L93 (-28.863, 46.6688, 84.7291) -> (-36.4777, 41.9594, 85.6701) construction
  line L94 (-36.4777, 41.9594, 85.6701) -> (-42.9101, 35.3544, 86.6111) construction
  line L95 (-42.9101, 35.3544, 86.6111) -> (-47.4163, 27.6178, 87.5522) construction
  line L96 (-47.4163, 27.6178, 87.5522) -> (-51.9224, 19.8813, 88.4932) construction
  line L97 (-51.9224, 19.8813, 88.4932) -> (-54.4939, 11.0279, 89.4342) construction
  line L98 (-54.4939, 11.0279, 89.4342) -> (-54.8335, 2.0812, 90.3752) construction
  line L99 (-54.8335, 2.0812, 90.3752) -> (-55.1731, -6.8652, 91.3162) construction
  line L100 (-55.1731, -6.8652, 91.3162) -> (-53.2802, -15.8879, 92.2572) construction
  line L101 (-53.2802, -15.8879, 92.2572) -> (-49.3736, -23.9435, 93.1982) construction
  line L102 (-49.3736, -23.9435, 93.1982) -> (-45.4672, -31.9989, 94.1391) construction
  line L103 (-45.4672, -31.9989, 94.1391) -> (-39.5547, -39.072, 95.0801) construction
  line L104 (-39.5547, -39.072, 95.0801) -> (-32.3197, -44.345, 96.021) construction
  line L105 (-32.3197, -44.345, 96.021) -> (-25.0849, -49.6179, 96.962) construction
  line L106 (-25.0849, -49.6179, 96.962) -> (-16.5414, -53.0808, 97.9029) construction
  line L107 (-16.5414, -53.0808, 97.9029) -> (-7.6771, -54.3333, 98.8438) construction
  line L108 (-7.6771, -54.3333, 98.8438) -> (1.187, -55.5858, 99.7848) construction
  line L109 (1.187, -55.5858, 99.7848) -> (10.3553, -54.6256, 100.7257) construction
  line L110 (10.3553, -54.6256, 100.7257) -> (18.7676, -51.5638, 101.6666) construction
  line L111 (18.7676, -51.5638, 101.6666) -> (27.5797, -48.3565, 102.6522) construction
  line L112 (27.5797, -48.3565, 102.6522) -> (35.542, -42.8457, 103.6378) construction
  line L113 (35.542, -42.8457, 103.6378) -> (41.6478, -35.7282, 104.6235) construction
  line L114 (41.6478, -35.7282, 104.6235) -> (47.706, -28.6663, 105.6014) construction
  line L115 (47.706, -28.6663, 105.6014) -> (51.9236, -20.039, 106.5793) construction
  line L116 (51.9236, -20.039, 106.5793) -> (53.7753, -10.9208, 107.5573) construction
  line L117 (53.7753, -10.9208, 107.5573) -> (55.6126, -1.8738, 108.5276) construction
  line L118 (55.6126, -1.8738, 108.5276) -> (55.1176, 7.6368, 109.4978) construction
  line L119 (55.1176, 7.6368, 109.4978) -> (52.3511, 16.4442, 110.4681) construction
  line L120 (52.3511, 16.4442, 110.4681) -> (49.6062, 25.1828, 111.4308) construction
  line L121 (49.6062, 25.1828, 111.4308) -> (44.6315, 33.211, 112.3935) construction
  line L122 (44.6315, 33.211, 112.3935) -> (38.0283, 39.5588, 113.3563) construction
  line L123 (38.0283, 39.5588, 113.3563) -> (31.4766, 45.857, 114.3114) construction
  line L124 (31.4766, 45.857, 114.3114) -> (23.3354, 50.4886, 115.2666) construction
  line L125 (23.3354, 50.4886, 115.2666) -> (14.5739, 52.9023, 116.2218) construction
  line L126 (14.5739, 52.9023, 116.2218) -> (5.8807, 55.2971, 117.1695) construction
  line L127 (5.8807, 55.2971, 117.1695) -> (-3.4059, 55.5045, 118.1173) construction
  line L128 (-3.4059, 55.5045, 118.1173) -> (-12.1973, 53.5002, 119.065) construction
  line L129 (-12.1973, 53.5002, 119.065) -> (-20.9635, 51.5016, 120.01) construction
  line L130 (-20.9635, 51.5016, 120.01) -> (-29.2203, 47.3081, 120.955) construction
  line L131 (-29.2203, 47.3081, 120.955) -> (-36.0052, 41.4086, 121.9) construction
  line L132 (-36.0052, 41.4086, 121.9) -> (-42.7894, 35.5096, 122.8449) construction
  line L133 (-42.7894, 35.5096, 122.8449) -> (-48.089, 27.9163, 123.7898) construction
  line L134 (-48.089, 27.9163, 123.7898) -> (-51.286, 19.5138, 124.7347) construction
  line L135 (-51.286, 19.5138, 124.7347) -> (-54.4828, 11.112, 125.6795) construction
  line L136 (-54.4828, 11.112, 125.6795) -> (-55.5714, 1.9174, 126.6244) construction
  line L137 (-55.5714, 1.9174, 126.6244) -> (-54.4249, -6.9986, 127.5692) construction
  line L138 (-54.4249, -6.9986, 127.5692) -> (-53.2785, -15.9137, 128.5139) construction
  line L139 (-53.2785, -15.9137, 128.5139) -> (-49.8996, -24.533, 129.4587) construction
  line L140 (-49.8996, -24.533, 129.4587) -> (-44.682, -31.8522, 130.4034) construction
  line L141 (-44.682, -31.8522, 130.4034) -> (-39.4649, -39.1707, 131.348) construction
  line L142 (-39.4649, -39.1707, 131.348) -> (-32.4194, -45.1753, 132.2927) construction